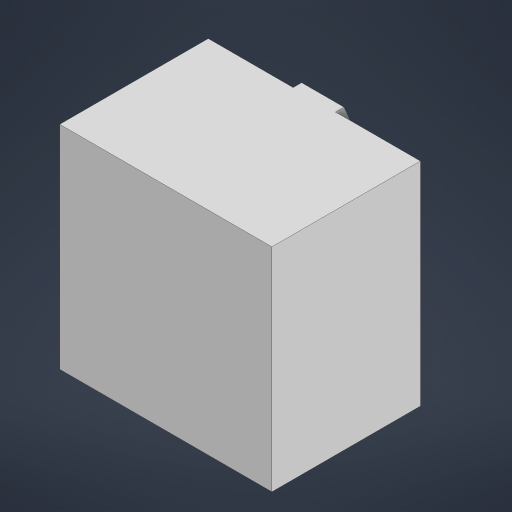
# Autodesk Inventor part: prueba
Saved by Autodesk Inventor 2024.1 (Build 281209000, 209)
## iProperties
Created: 2023-07-19
Part Number: prueba
Material: Generic
Document SubType Name: Modeling
Designer: LabTel_Admin
Density: 1 g/cm^3
Appearance: Default
Author: LabTel_Admin
Autodesk Inventor part; units mm, degrees
ref_plane "YZ Plane" through (0, 0, 0) normal (1, 0, 0) x (0, 1, 0)
ref_plane "XZ Plane" through (0, 0, 0) normal (0, 1, 0) x (-1, 0, 0)
ref_plane "XY Plane" through (0, 0, 0) normal (0, 0, 1) x (1, 0, 0)
sketch "Sketch1" plane through (0, 0, 0) normal (0, 1, 0) x (-1, 0, 0)
  line L0 (0, 0) -> (-10, 0)
  line L1 (-10, 0) -> (-10, -7)
  line L2 (-10, -7) -> (0, -7)
  line L3 (0, -7) -> (0, 0)
  dimension "d0" = 10
  dimension "d1" = 7
  constraints: 8 end point, 2 parallel, 1 horizontal, 1 perpendicular
  measures "d0" distance of L2.end L1.end
  measures "d1" distance of L1.end L0.end
extrude "Extrusion1" add sketch "Sketch1" along normal blind 10
sketch "Sketch2" plane through (10, 0, -7) normal (0, 0, -1) x (-1, 0, 0)
  line L0 (0, 10) -> (10, 10) projected
  line L1 (4, 10) -> (6, 10)
  line L2 (6, 10) -> (6, 7)
  line L3 (6, 7) -> (4, 7)
  line L4 (4, 7) -> (4, 10)
  line L5 (10, 0) -> (10, 10) projected
  dimension "d4" = 2
  dimension "d5" = 3
  dimension "d6" = 4
  constraints: 8 end point, 2 parallel, 1 horizontal, 1 perpendicular, 1 point on line
  measures "d4" distance of L2.end L3.end
  measures "d5" distance of L1.end L2.end
  measures "d6" distance between parallel lines of L5 L2
extrude "Extrusion2" add sketch "Sketch2" along normal blind 1.5
sketch "Sketch3" plane through (6, 7, -7) normal (1, 0, 0) x (0, 0, -1)
  line L0 (0, 3) -> (1.5, 3) projected
  line L1 (0.4, 3) -> (1.5, 0.4)
  line L2 (1.5, 0) -> (1.5, 3) projected
  line L3 (0, -7) -> (0, 3) projected
  line L4 (0, 0) -> (1.5, 0) projected
  line L5 (0.4, 3) -> (1.5, 3)
  line L6 (1.5, 0.4) -> (1.5, 3)
  point P0 (-7, -7)
  dimension "d9" = 0.4
  dimension "d10" = 0.4
  constraints: 6 end point, 2 collinear, 2 point on line
  measures "d9" distance from line of L3 L1.start
  measures "d10" distance from line of L4 L1.end
extrude "Extrusion3" cut sketch "Sketch3" against normal through all contours L0 L2 L1
body "Solid1"
